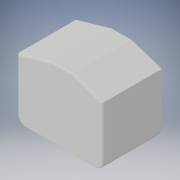
# Autodesk Inventor part: SCALE HEAD
Saved by Autodesk Inventor 2018 (Build 220112000, 112)
## iProperties
Created: 2018-05-04
Part Number: SCALE HEAD
Material: Generic
Document SubType Name: Modeling
Designer: 4070609
Density: 1 g/cm^3
Appearance: Default
Author: 4070609
Autodesk Inventor part; units mm, degrees
ref_plane "YZ Plane" through (0, 0, 0) normal (1, 0, 0) x (0, 1, 0)
ref_plane "XZ Plane" through (0, 0, 0) normal (0, 1, 0) x (-1, 0, 0)
ref_plane "XY Plane" through (0, 0, 0) normal (0, 0, 1) x (1, 0, 0)
sketch "Sketch1" plane through (0, 0, 0) normal (0, 0, 1) x (1, 0, 0)
  line L0 (0, 0) -> (85, 0)
  line L1 (85, 0) -> (85, 60)
  line L2 (85, 60) -> (0, 60)
  line L3 (0, 60) -> (0, 0)
  line L4 (0, 60) -> (35, 60)
  line L5 (35, 60) -> (35, 70)
  line L6 (35, 70) -> (55, 70)
  line L7 (55, 70) -> (85, 60)
  line L8 (35, 70) -> (0, 60)
  dimension "d0" = 85
  dimension "d1" = 60
  dimension "d2" = 35
  dimension "d3" = 10
  dimension "d4" = 20
  constraints: 18 end point, 2 horizontal, 2 parallel, 1 perpendicular, 1 point on line, 1 vertical
  measures "d0" distance of L2.end L1.end
  measures "d1" distance of L1.end L0.end
  measures "d2" distance of L2.end L4.end
  measures "d3" distance of L4.end L5.end
  measures "d4" distance of L5.end L6.end
extrude "Extrusion1" add sketch "Sketch1" along normal blind 60
fillet "Fillet1" radius 8 2 edges at (85, 0, 30) (0, 0, 30)
fillet "Fillet2" radius 2 16 edges at (82.6569, 2.3431, 60) (42.5, 0, 60) (2.3431, 2.3431, 60) (0, 34, 60) (85, 34, 60) (70, 65, 60) (45, 70, 60) (17.5, 65, 60) (82.6569, 2.3431, 0) (42.5, 0, 0) (2.3431, 2.3431, 0) (0, 34, 0) (85, 34, 0) (70, 65, 0) (45, 70, 0) (17.5, 65, 0)
sketch "Sketch2" plane through (0, 0, 0) normal (0, 0, -1) x (-1, 0, 0)
  point P0 (0, 0)
sketch "Sketch3" plane through (0, 0, 0) normal (0, 0, -1) x (-1, 0, 0)
  line L0 (-85, 8) -> (-85, 60) projected
  circle A0 centre (-27.9194, 43) radius 7.5
  circle A1 centre (-56.1406, 43) radius 7.5
  point P0 (0, 0)
  dimension "d12" = 15
  constraints: 2 centre point
  measures "d12" diameter of A0
extrude "Extrusion2" cut sketch "Sketch3" against normal blind 5
body "Solid1"
